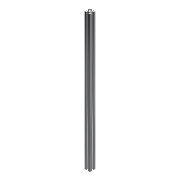
# Autodesk Inventor part: HFS5-2020
Saved by Autodesk Inventor 2018.2 (Build 222227000, 227)
## iProperties
Created: 2015-06-02
Part Number: HFS5-2020
Material: Aluminum 6061
Document SubType Name: Modeling
Designer: Sawaiz Syed
Density: 2.7 g/cm^3
Appearance: Aluminum - Flat
Author: Sawaiz Syed
Autodesk Inventor part; units mm, degrees
ref_plane "YZ Plane" through (0, 0, 0) normal (1, 0, 0) x (0, 1, 0)
ref_plane "XZ Plane" through (0, 0, 0) normal (0, 1, 0) x (-1, 0, 0)
ref_plane "XY Plane" through (0, 0, 0) normal (0, 0, 1) x (1, 0, 0)
sketch "Sketch1" plane through (0, 0, 0) normal (0, 0, 1) x (1, 0, 0)
  line L0 (-2.205, 0) -> (2.205, 0)
  line L1 (0, -2.205) -> (0, 2.205)
  arc A0 (9, -10) -> (10, -9) centre (9, -9) ccw
  line L2 (-10, 9) -> (-10, 3)
  line L3 (-10, 3) -> (-8, 3)
  line L4 (-8, 3) -> (-8, 6)
  line L5 (-8, 6) -> (-7.0607, 6)
  line L6 (-7.0607, 6) -> (-4, 2.9393)
  line L7 (-4, 2.9393) -> (-4, 0.5196)
  line L8 (-4, 0.5196) -> (-3.7, 0)
  line L9 (-3.7, 0) -> (-4, -0.5196)
  line L10 (-4, -0.5196) -> (-4, -2.9393)
  line L11 (-4, -2.9393) -> (-7.0607, -6)
  line L12 (-7.0607, -6) -> (-8, -6)
  line L13 (-8, -6) -> (-8, -3)
  line L14 (-8, -3) -> (-10, -3)
  line L15 (-10, -3) -> (-10, -9)
  arc A1 (-10, -9) -> (-9, -10) centre (-9, -9) ccw
  line L16 (-9, -10) -> (-3, -10)
  line L17 (-3, -10) -> (-3, -8)
  line L18 (-3, -8) -> (-6, -8)
  line L19 (-6, -7.0607) -> (-2.9393, -4)
  line L20 (-2.9393, -4) -> (-0.5196, -4)
  line L21 (-0.5196, -4) -> (0, -3.7)
  line L22 (0, -3.7) -> (0.5196, -4)
  line L23 (0.5196, -4) -> (2.9393, -4)
  line L24 (2.9393, -4) -> (6, -7.0607)
  line L25 (6, -7.0607) -> (6, -8)
  line L26 (6, -8) -> (3, -8)
  line L27 (3, -8) -> (3, -10)
  line L28 (3, -10) -> (9, -10)
  line L29 (10, -9) -> (10, -3)
  line L30 (10, -3) -> (8, -3)
  line L31 (8, -3) -> (8, -6)
  line L32 (8, -6) -> (7.0607, -6)
  line L33 (7.0607, -6) -> (4, -2.9393)
  line L34 (4, -2.9393) -> (4, -0.5196)
  line L35 (4, -0.5196) -> (3.7, 0)
  line L36 (3.7, 0) -> (4, 0.5196)
  line L37 (4, 0.5196) -> (4, 2.9393)
  line L38 (4, 2.9393) -> (7.0607, 6)
  line L39 (7.0607, 6) -> (8, 6)
  line L40 (8, 6) -> (8, 3)
  line L41 (8, 3) -> (10, 3)
  line L42 (10, 3) -> (10, 9)
  arc A2 (10, 9) -> (9, 10) centre (9, 9) ccw
  line L43 (9, 10) -> (3, 10)
  line L44 (3, 10) -> (3, 8)
  line L45 (3, 8) -> (6, 8)
  line L46 (6, 8) -> (6, 7.0607)
  line L47 (6, 7.0607) -> (2.9393, 4)
  line L48 (2.9393, 4) -> (0.5196, 4)
  line L49 (0.5196, 4) -> (0, 3.7)
  line L50 (0, 3.7) -> (-0.5196, 4)
  line L51 (-0.5196, 4) -> (-2.9393, 4)
  line L52 (-2.9393, 4) -> (-6, 7.0607)
  line L53 (-6, 7.0607) -> (-6, 8)
  line L54 (-6, 8) -> (-3, 8)
  line L55 (-3, 8) -> (-3, 10)
  line L56 (-3, 10) -> (-9, 10)
  arc A3 (-9, 10) -> (-10, 9) centre (-9, 9) ccw
  circle A4 centre (0, 0) radius 2.1
  line L57 (-6, -8) -> (-6, -7.0607)
  constraints: 116 end point, 8 point on circle, 5 centre point, 1 coincident
extrude "Extrusion1" add sketch "Sketch1" along normal mid plane 500
equation "\"d0\" = depth"
equation "\"depth\" = 500"
body "Solid1"
